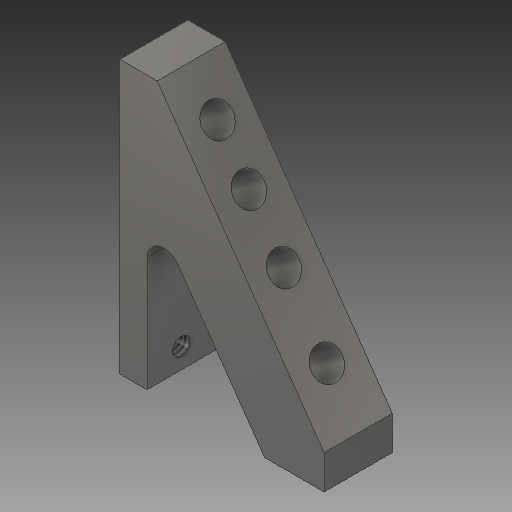
# Autodesk Inventor part: Punch Holder
Saved by Autodesk Inventor 2018 (Build 220112000, 112)
## iProperties
Created: 2017-12-21
Part Number: Punch Holder
Material: Stainless Steel
Document SubType Name: Modeling
Designer: 232963
Density: 8 g/cm^3
Appearance: Semi-Polished
Author: 232963
Autodesk Inventor part; units mm, degrees
ref_plane "YZ Plane" through (0, 0, 0) normal (1, 0, 0) x (0, 1, 0)
ref_plane "XZ Plane" through (0, 0, 0) normal (0, 1, 0) x (-1, 0, 0)
ref_plane "XY Plane" through (0, 0, 0) normal (0, 0, 1) x (1, 0, 0)
sketch "Sketch1" plane through (0, 0, 0) normal (0, 0, 1) x (1, 0, 0)
  line L0 (-12.8542, 0) -> (25.2458, 0)
  line L1 (25.2458, 0) -> (25.2458, 50.8)
  line L2 (25.2458, 50.8) -> (-12.8542, 50.8)
  line L3 (-12.8542, 50.8) -> (-12.8542, 0)
  circle A0 centre (-4.5992, 21.2852) radius 3.175
  line L4 (-7.7742, 21.2852) -> (-7.7742, 0)
  line L5 (-1.9984, 23.1063) -> (14.1808, 0)
  line L6 (-5.8785, 50.8) -> (25.2458, 6.35)
  point P0 (0, 0)
  dimension "d0" = 38.1
  dimension "d1" = 50.8
  dimension "d2" = 6.35
  dimension "d3" = 8.255
  dimension "d4" = 21.2852
  dimension "d5" = 6.35
  dimension "d6" = 35
  constraints: 14 end point, 4 point on line, 3 parallel, 2 perpendicular, 2 point on circle, 2 tangent, 1 centre point, 1 horizontal
  measures "d0" distance of L2.end L1.end
  measures "d1" distance of L1.end L0.end
  measures "d2" diameter of A0
  measures "d3" distance from line of L3 A0.centre
  measures "d4" distance from line of L0 A0.centre
  measures "d5" distance from line of L0 L6.end
  measures "d6" angle of L3 L6
extrude "Extrusion1" add sketch "Sketch1" along normal blind 12.7 contours L3 L2 L6 L1 L0 L5 A0 L4
sketch "Sketch2" plane through (-5.8785, 50.8, 12.7) normal (0.819152, 0.5735764, 0) x (0, 0, -1)
  circle A0 centre (6.35, -8.5344) radius 2.8702
  circle A1 centre (6.35, -18.6944) radius 2.8702
  circle A2 centre (6.35, -30.1244) radius 2.8702
  circle A3 centre (6.35, -44.0944) radius 2.8702
  line L0 (12.7, 0) -> (0, 0) projected
  line L1 (12.7, -54.2634) -> (12.7, 0) projected
  point P0 (12.7, -44.9847)
  dimension "d9" = 5.7404
  dimension "d10" = 5.7404
  dimension "d11" = 5.7404
  dimension "d12" = 5.7404
  dimension "d13" = 8.5344
  dimension "d14" = 6.35
  dimension "d16" = 30.1244
  dimension "d17" = 44.0944
  dimension "d18" = 18.6944
  constraints: 4 centre point, 4 vertical alignment
  measures "d9" diameter of A0
  measures "d10" diameter of A1
  measures "d11" diameter of A2
  measures "d12" diameter of A3
  measures "d13" distance from line of L0 A0.centre
  measures "d14" distance from line of L1 A0.centre
  measures "d16" distance from line of L0 A2.centre
  measures "d17" distance from line of L0 A3.centre
  measures "d18" distance from line of L0 A1.centre
extrude "Extrusion2" cut sketch "Sketch2" against normal blind 10.16
sketch "Sketch3" plane through (-12.8542, 0, 0) normal (-1, 0, 0) x (0, 0, 1)
  line L0 (0, 50.8) -> (0, 0) projected
  line L1 (0, 0) -> (12.7, 0) projected
  point P0 (6.35, 46.99)
  point P1 (6.35, 3.81)
  dimension "d21" = 6.35
  dimension "d22" = 6.35
  dimension "d23" = 46.99
  dimension "d24" = 3.81
  measures "d21" distance from line of L0 point (6.35, 46.99)
  measures "d22" distance from line of L0 point (6.35, 3.81)
  measures "d23" distance from line of L1 point (6.35, 46.99)
  measures "d24" distance from line of L1 point (6.35, 3.81)
hole "Hole1" at (-12.8542, 46.99, 6.35) at (-12.8542, 3.81, 6.35) direction (1, 0, 0) diameter 3.302 depth 7.62 tip angle 118 thread size "8-32 UNC" class "2B" standard "ANSI Unified Screw Threads"
equation "\"d10\" = d9"
equation "\"d11\" = d9"
equation "\"d12\" = d9"
body "Solid1"
